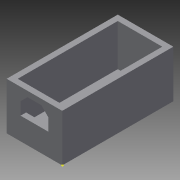
# Autodesk Inventor part: nano_enclosure
Saved by Autodesk Inventor 2015 (Build 190159000, 159)
## iProperties
Created: 2015-02-05
Part Number: nano_enclosure
Material: Generic
Document SubType Name: Modeling
Designer: Jeff
Density: 1 g/cm^3
Appearance: Default
Author: Jeff
Autodesk Inventor part; units mm, degrees
ref_plane "YZ Plane" through (0, 0, 0) normal (1, 0, 0) x (0, 1, 0)
ref_plane "XZ Plane" through (0, 0, 0) normal (0, 1, 0) x (-1, 0, 0)
ref_plane "XY Plane" through (0, 0, 0) normal (0, 0, 1) x (1, 0, 0)
sketch "Sketch1" plane through (0, 0, 0) normal (0, 1, 0) x (-1, 0, 0)
  line L0 (0, 0) -> (25.4, 0)
  line L1 (25.4, 0) -> (25.4, -50.8)
  line L2 (25.4, -50.8) -> (0, -50.8)
  line L3 (0, -50.8) -> (0, 0)
  dimension "d0" = 25.4
  dimension "d1" = 50.8
  constraints: 8 end point, 2 parallel, 1 horizontal, 1 perpendicular
  measures "d0" distance of L1.end L2.end
  measures "d1" distance of L0.end L1.end
extrude "Extrusion1" add sketch "Sketch1" along normal blind 21.59
shell "Shell1" thickness 2.54 removed faces 1 at (-8.4667, 21.59, -33.8667)
sketch "Sketch3" plane through (-25.4, 0, 0) normal (0, 0, 1) x (1, 0, 0)
  line L0 (19.05, 10.16) -> (6.35, 10.16)
  line L1 (6.35, 10.16) -> (6.35, 19.05)
  line L2 (6.35, 19.05) -> (19.05, 19.05)
  line L3 (19.05, 19.05) -> (19.05, 10.16)
  point P0 (25.4, 0)
  dimension "d20" = 10.16
  dimension "d21" = 12.7
  dimension "d22" = 8.89
  dimension "d23" = 6.35
  constraints: 8 end point, 2 parallel, 1 horizontal, 1 perpendicular
  measures "d20" distance from line of point (25.4, 0) L0
  measures "d21" distance of L1.end L2.end
  measures "d22" distance of L2.end L0.start
  measures "d23" distance from line of point (25.4, 0) L3
extrude "Extrusion3" cut sketch "Sketch3" against normal blind 2.54
chamfer "Chamfer1" distance 3.175 angle 45 2 edges at (-19.05, 19.05, -1.27) (-6.35, 19.05, -1.27)
body "Solid1"
